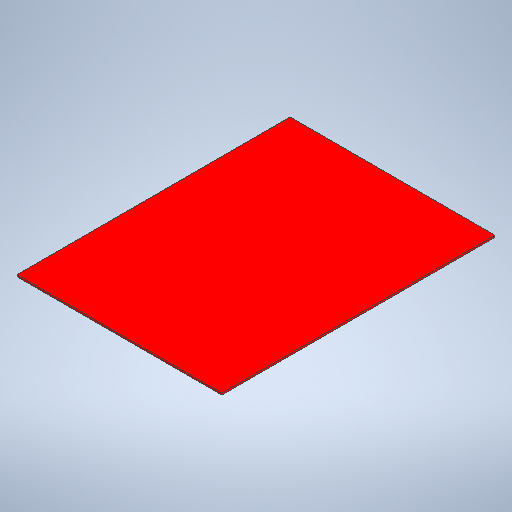
# Autodesk Inventor part: thermal pad
Saved by Autodesk Inventor 2025.2 (Build 292293000, 293)
## iProperties
Created: 2024-11-29
Part Number: thermal pad
Material: Generic
Document SubType Name: Modeling
Designer: cbast
Density: 1 g/cm^3
Appearance: Default
Author: cbast
Autodesk Inventor part; units mm, degrees
ref_plane "YZ Plane" through (0, 0, 0) normal (1, 0, 0) x (0, 1, 0)
ref_plane "XZ Plane" through (0, 0, 0) normal (0, 1, 0) x (-1, 0, 0)
ref_plane "XY Plane" through (0, 0, 0) normal (0, 0, 1) x (1, 0, 0)
sketch "Sketch1" plane through (0, 0, 0) normal (0, 1, 0) x (-1, 0, 0)
  line L0 (57.15, 128.6605) -> (-57.15, 128.6605)
  line L1 (-57.15, 128.6605) -> (-57.15, -23.7395)
  line L2 (-57.15, -23.7395) -> (57.15, -23.7395)
  line L3 (57.15, -23.7395) -> (57.15, 128.6605)
  line L4 (57.15, 128.6605) -> (-57.15, -23.7395) construction
  line L5 (-57.15, 128.6605) -> (57.15, -23.7395) construction
  point P0 (0, 52.4605)
  dimension "d7" = 114.3
  dimension "d8" = 152.4
  constraints: 12 end point, 2 midpoint, 2 parallel, 1 horizontal, 1 perpendicular
  measures "d7" distance of L2.end L1.end
  measures "d8" distance of L0.end L1.end
extrude "Extrusion1" add sketch "Sketch1" along normal blind 1
body "Solid1"
